Autodesk Fusion 360 part; units mm, degrees
(part 7 of 14)
  line L3871 (218.2079, 114.3) -> (223.7072, 123.825)
  line L3872 (237.4553, 144.4625) -> (226.4568, 144.4625)
  line L3873 (226.4568, 144.4625) -> (220.9575, 134.9375)
  line L3874 (220.9575, 134.9375) -> (226.4568, 125.4125)
  line L3875 (226.4568, 125.4125) -> (237.4553, 125.4125)
  line L3876 (242.9546, 134.9375) -> (237.4553, 144.4625)
  line L3877 (237.4553, 125.4125) -> (242.9546, 134.9375)
  line L3878 (256.7027, 155.575) -> (245.7042, 155.575)
  line L3879 (245.7042, 155.575) -> (240.2049, 146.05)
  line L3880 (240.2049, 146.05) -> (245.7042, 136.525)
  line L3881 (245.7042, 136.525) -> (256.7027, 136.525)
  line L3882 (262.202, 146.05) -> (256.7027, 155.575)
  line L3883 (256.7027, 136.525) -> (262.202, 146.05)
  line L3884 (275.9501, 166.6875) -> (264.9516, 166.6875)
  line L3885 (264.9516, 166.6875) -> (259.4524, 157.1625)
  line L3886 (259.4524, 157.1625) -> (264.9516, 147.6375)
  line L3887 (264.9516, 147.6375) -> (275.9501, 147.6375)
  line L3888 (281.4494, 157.1625) -> (275.9501, 166.6875)
  line L3889 (275.9501, 147.6375) -> (281.4494, 157.1625)
  line L3890 (295.1976, 177.8) -> (284.199, 177.8)
  line L3891 (284.199, 177.8) -> (278.6998, 168.275)
  line L3892 (278.6998, 168.275) -> (284.199, 158.75)
  line L3893 (284.199, 158.75) -> (295.1976, 158.75)
  line L3894 (300.6968, 168.275) -> (295.1976, 177.8)
  line L3895 (295.1976, 158.75) -> (300.6968, 168.275)
  line L3896 (314.445, 188.9125) -> (303.4464, 188.9125)
  line L3897 (303.4464, 188.9125) -> (297.9472, 179.3875)
  line L3898 (297.9472, 179.3875) -> (303.4464, 169.8625)
  line L3899 (303.4464, 169.8625) -> (314.445, 169.8625)
  line L3900 (319.9442, 179.3875) -> (314.445, 188.9125)
  line L3901 (314.445, 169.8625) -> (319.9442, 179.3875)
  line L3902 (333.6924, 200.025) -> (322.6939, 200.025)
  line L3903 (322.6939, 200.025) -> (317.1946, 190.5)
  line L3904 (317.1946, 190.5) -> (322.6939, 180.975)
  line L3905 (322.6939, 180.975) -> (333.6924, 180.975)
  line L3906 (339.1916, 190.5) -> (333.6924, 200.025)
  line L3907 (333.6924, 180.975) -> (339.1916, 190.5)
  line L3908 (352.9398, 211.1375) -> (341.9413, 211.1375)
  line L3909 (341.9413, 211.1375) -> (336.442, 201.6125)
  line L3910 (336.442, 201.6125) -> (341.9413, 192.0875)
  line L3911 (341.9413, 192.0875) -> (352.9398, 192.0875)
  line L3912 (358.4391, 201.6125) -> (352.9398, 211.1375)
  line L3913 (352.9398, 192.0875) -> (358.4391, 201.6125)
  line L3914 (372.1872, 222.25) -> (361.1887, 222.25)
  line L3915 (361.1887, 222.25) -> (355.6894, 212.725)
  line L3916 (355.6894, 212.725) -> (361.1887, 203.2)
  line L3917 (361.1887, 203.2) -> (372.1872, 203.2)
  line L3918 (377.6865, 212.725) -> (372.1872, 222.25)
  line L3919 (372.1872, 203.2) -> (377.6865, 212.725)
  line L3920 (391.4346, 233.3625) -> (380.4361, 233.3625)
  line L3921 (380.4361, 233.3625) -> (374.9368, 223.8375)
  line L3922 (374.9368, 223.8375) -> (380.4361, 214.3125)
  line L3923 (380.4361, 214.3125) -> (391.4346, 214.3125)
  line L3924 (396.9339, 223.8375) -> (391.4346, 233.3625)
  line L3925 (391.4346, 214.3125) -> (396.9339, 223.8375)
  line L3926 (410.682, 244.475) -> (399.6835, 244.475)
  line L3927 (399.6835, 244.475) -> (394.1843, 234.95)
  line L3928 (394.1843, 234.95) -> (399.6835, 225.425)
  line L3929 (399.6835, 225.425) -> (410.682, 225.425)
  line L3930 (416.1813, 234.95) -> (410.682, 244.475)
  line L3931 (410.682, 225.425) -> (416.1813, 234.95)
  line L3932 (429.9295, 255.5875) -> (418.9309, 255.5875)
  line L3933 (418.9309, 255.5875) -> (413.4317, 246.0625)
  line L3934 (413.4317, 246.0625) -> (418.9309, 236.5375)
  line L3935 (418.9309, 236.5375) -> (429.9295, 236.5375)
  line L3936 (435.4287, 246.0625) -> (429.9295, 255.5875)
  line L3937 (429.9295, 236.5375) -> (435.4287, 246.0625)
  line L3938 (449.1769, 266.7) -> (438.1783, 266.7)
  line L3939 (438.1783, 266.7) -> (432.6791, 257.175)
  line L3940 (432.6791, 257.175) -> (438.1783, 247.65)
  line L3941 (438.1783, 247.65) -> (449.1769, 247.65)
  line L3942 (454.6761, 257.175) -> (449.1769, 266.7)
  line L3943 (449.1769, 247.65) -> (454.6761, 257.175)
  line L3944 (468.4243, 277.8125) -> (457.4258, 277.8125)
  line L3945 (457.4258, 277.8125) -> (451.9265, 268.2875)
  line L3946 (451.9265, 268.2875) -> (457.4258, 258.7625)
  line L3947 (457.4258, 258.7625) -> (468.4243, 258.7625)
  line L3948 (473.9235, 268.2875) -> (468.4243, 277.8125)
  line L3949 (468.4243, 258.7625) -> (473.9235, 268.2875)
  line L3950 (487.6717, 288.925) -> (476.6732, 288.925)
  line L3951 (476.6732, 288.925) -> (471.1739, 279.4)
  line L3952 (471.1739, 279.4) -> (476.6732, 269.875)
  line L3953 (476.6732, 269.875) -> (487.6717, 269.875)
  line L3954 (493.171, 279.4) -> (487.6717, 288.925)
  line L3955 (487.6717, 269.875) -> (493.171, 279.4)
  line L3956 (506.9191, 300.0375) -> (495.9206, 300.0375)
  line L3957 (495.9206, 300.0375) -> (490.4213, 290.5125)
  line L3958 (490.4213, 290.5125) -> (495.9206, 280.9875)
  line L3959 (495.9206, 280.9875) -> (506.9191, 280.9875)
  line L3960 (512.4184, 290.5125) -> (506.9191, 300.0375)
  line L3961 (506.9191, 280.9875) -> (512.4184, 290.5125)
  line L3962 (526.1665, 311.15) -> (515.168, 311.15)
  line L3963 (515.168, 311.15) -> (509.6687, 301.625)
  line L3964 (509.6687, 301.625) -> (515.168, 292.1)
  line L3965 (515.168, 292.1) -> (526.1665, 292.1)
  line L3966 (531.6658, 301.625) -> (526.1665, 311.15)
  line L3967 (526.1665, 292.1) -> (531.6658, 301.625)
  line L3968 (545.4139, 322.2625) -> (534.4154, 322.2625)
  line L3969 (534.4154, 322.2625) -> (528.9162, 312.7375)
  line L3970 (528.9162, 312.7375) -> (534.4154, 303.2125)
  line L3971 (534.4154, 303.2125) -> (545.4139, 303.2125)
  line L3972 (550.9132, 312.7375) -> (545.4139, 322.2625)
  line L3973 (545.4139, 303.2125) -> (550.9132, 312.7375)
  line L3974 (564.6614, 333.375) -> (553.6628, 333.375)
  line L3975 (553.6628, 333.375) -> (548.1636, 323.85)
  line L3976 (548.1636, 323.85) -> (553.6628, 314.325)
  line L3977 (553.6628, 314.325) -> (564.6614, 314.325)
  line L3978 (570.1606, 323.85) -> (564.6614, 333.375)
  line L3979 (564.6614, 314.325) -> (570.1606, 323.85)
  line L3980 (-590.1835, -311.15) -> (-601.182, -311.15)
  line L3981 (-601.182, -311.15) -> (-606.6813, -320.675)
  line L3982 (-606.6813, -320.675) -> (-601.182, -330.2)
  line L3983 (-601.182, -330.2) -> (-590.1835, -330.2)
  line L3984 (-584.6843, -320.675) -> (-590.1835, -311.15)
  line L3985 (-590.1835, -330.2) -> (-584.6843, -320.675)
  line L3986 (-570.9361, -300.0375) -> (-581.9346, -300.0375)
  line L3987 (-581.9346, -300.0375) -> (-587.4339, -309.5625)
  line L3988 (-587.4339, -309.5625) -> (-581.9346, -319.0875)
  line L3989 (-581.9346, -319.0875) -> (-570.9361, -319.0875)
  line L3990 (-565.4368, -309.5625) -> (-570.9361, -300.0375)
  line L3991 (-570.9361, -319.0875) -> (-565.4368, -309.5625)
  line L3992 (-551.6887, -288.925) -> (-562.6872, -288.925)
  line L3993 (-562.6872, -288.925) -> (-568.1865, -298.45)
  line L3994 (-568.1865, -298.45) -> (-562.6872, -307.975)
  line L3995 (-562.6872, -307.975) -> (-551.6887, -307.975)
  line L3996 (-546.1894, -298.45) -> (-551.6887, -288.925)
  line L3997 (-551.6887, -307.975) -> (-546.1894, -298.45)
  line L3998 (-532.4413, -277.8125) -> (-543.4398, -277.8125)
  line L3999 (-543.4398, -277.8125) -> (-548.9391, -287.3375)
  line L4000 (-548.9391, -287.3375) -> (-543.4398, -296.8625)
  line L4001 (-543.4398, -296.8625) -> (-532.4413, -296.8625)
  line L4002 (-526.942, -287.3375) -> (-532.4413, -277.8125)
  line L4003 (-532.4413, -296.8625) -> (-526.942, -287.3375)
  line L4004 (-513.1939, -266.7) -> (-524.1924, -266.7)
  line L4005 (-524.1924, -266.7) -> (-529.6916, -276.225)
  line L4006 (-529.6916, -276.225) -> (-524.1924, -285.75)
  line L4007 (-524.1924, -285.75) -> (-513.1939, -285.75)
  line L4008 (-507.6946, -276.225) -> (-513.1939, -266.7)
  line L4009 (-513.1939, -285.75) -> (-507.6946, -276.225)
  line L4010 (-493.9464, -255.5875) -> (-504.945, -255.5875)
  line L4011 (-504.945, -255.5875) -> (-510.4442, -265.1125)
  line L4012 (-510.4442, -265.1125) -> (-504.945, -274.6375)
  line L4013 (-504.945, -274.6375) -> (-493.9464, -274.6375)
  line L4014 (-488.4472, -265.1125) -> (-493.9464, -255.5875)
  line L4015 (-493.9464, -274.6375) -> (-488.4472, -265.1125)
  line L4016 (-474.699, -244.475) -> (-485.6976, -244.475)
  line L4017 (-485.6976, -244.475) -> (-491.1968, -254)
  line L4018 (-491.1968, -254) -> (-485.6976, -263.525)
  line L4019 (-485.6976, -263.525) -> (-474.699, -263.525)
  line L4020 (-469.1998, -254) -> (-474.699, -244.475)
  line L4021 (-474.699, -263.525) -> (-469.1998, -254)
  line L4022 (-455.4516, -233.3625) -> (-466.4501, -233.3625)
  line L4023 (-466.4501, -233.3625) -> (-471.9494, -242.8875)
  line L4024 (-471.9494, -242.8875) -> (-466.4501, -252.4125)
  line L4025 (-466.4501, -252.4125) -> (-455.4516, -252.4125)
  line L4026 (-449.9524, -242.8875) -> (-455.4516, -233.3625)
  line L4027 (-455.4516, -252.4125) -> (-449.9524, -242.8875)
  line L4028 (-436.2042, -222.25) -> (-447.2027, -222.25)
  line L4029 (-447.2027, -222.25) -> (-452.702, -231.775)
  line L4030 (-452.702, -231.775) -> (-447.2027, -241.3)
  line L4031 (-447.2027, -241.3) -> (-436.2042, -241.3)
  line L4032 (-430.7049, -231.775) -> (-436.2042, -222.25)
  line L4033 (-436.2042, -241.3) -> (-430.7049, -231.775)
  line L4034 (-416.9568, -211.1375) -> (-427.9553, -211.1375)
  line L4035 (-427.9553, -211.1375) -> (-433.4546, -220.6625)
  line L4036 (-433.4546, -220.6625) -> (-427.9553, -230.1875)
  line L4037 (-427.9553, -230.1875) -> (-416.9568, -230.1875)
  line L4038 (-411.4575, -220.6625) -> (-416.9568, -211.1375)
  line L4039 (-416.9568, -230.1875) -> (-411.4575, -220.6625)
  line L4040 (-397.7094, -200.025) -> (-408.7079, -200.025)
  line L4041 (-408.7079, -200.025) -> (-414.2072, -209.55)
  line L4042 (-414.2072, -209.55) -> (-408.7079, -219.075)
  line L4043 (-408.7079, -219.075) -> (-397.7094, -219.075)
  line L4044 (-392.2101, -209.55) -> (-397.7094, -200.025)
  line L4045 (-397.7094, -219.075) -> (-392.2101, -209.55)
  line L4046 (-378.462, -188.9125) -> (-389.4605, -188.9125)
  line L4047 (-389.4605, -188.9125) -> (-394.9597, -198.4375)
  line L4048 (-394.9597, -198.4375) -> (-389.4605, -207.9625)
  line L4049 (-389.4605, -207.9625) -> (-378.462, -207.9625)
  line L4050 (-372.9627, -198.4375) -> (-378.462, -188.9125)
  line L4051 (-378.462, -207.9625) -> (-372.9627, -198.4375)
  line L4052 (-359.2145, -177.8) -> (-370.2131, -177.8)
  line L4053 (-370.2131, -177.8) -> (-375.7123, -187.325)
  line L4054 (-375.7123, -187.325) -> (-370.2131, -196.85)
  line L4055 (-370.2131, -196.85) -> (-359.2145, -196.85)
  line L4056 (-353.7153, -187.325) -> (-359.2145, -177.8)
  line L4057 (-359.2145, -196.85) -> (-353.7153, -187.325)
  line L4058 (-339.9671, -166.6875) -> (-350.9657, -166.6875)
  line L4059 (-350.9657, -166.6875) -> (-356.4649, -176.2125)
  line L4060 (-356.4649, -176.2125) -> (-350.9657, -185.7375)
  line L4061 (-350.9657, -185.7375) -> (-339.9671, -185.7375)
  line L4062 (-334.4679, -176.2125) -> (-339.9671, -166.6875)
  line L4063 (-339.9671, -185.7375) -> (-334.4679, -176.2125)
  line L4064 (-320.7197, -155.575) -> (-331.7182, -155.575)
  line L4065 (-331.7182, -155.575) -> (-337.2175, -165.1)
  line L4066 (-337.2175, -165.1) -> (-331.7182, -174.625)
  line L4067 (-331.7182, -174.625) -> (-320.7197, -174.625)
  line L4068 (-315.2205, -165.1) -> (-320.7197, -155.575)
  line L4069 (-320.7197, -174.625) -> (-315.2205, -165.1)
  line L4070 (-301.4723, -144.4625) -> (-312.4708, -144.4625)
  line L4071 (-312.4708, -144.4625) -> (-317.9701, -153.9875)
  line L4072 (-317.9701, -153.9875) -> (-312.4708, -163.5125)
  line L4073 (-312.4708, -163.5125) -> (-301.4723, -163.5125)
  line L4074 (-295.973, -153.9875) -> (-301.4723, -144.4625)
  line L4075 (-301.4723, -163.5125) -> (-295.973, -153.9875)
  line L4076 (-282.2249, -133.35) -> (-293.2234, -133.35)
  line L4077 (-293.2234, -133.35) -> (-298.7227, -142.875)
  line L4078 (-298.7227, -142.875) -> (-293.2234, -152.4)
  line L4079 (-293.2234, -152.4) -> (-282.2249, -152.4)
  line L4080 (-276.7256, -142.875) -> (-282.2249, -133.35)
  line L4081 (-282.2249, -152.4) -> (-276.7256, -142.875)
  line L4082 (-262.9775, -122.2375) -> (-273.976, -122.2375)
  line L4083 (-273.976, -122.2375) -> (-279.4753, -131.7625)
  line L4084 (-279.4753, -131.7625) -> (-273.976, -141.2875)
  line L4085 (-273.976, -141.2875) -> (-262.9775, -141.2875)
  line L4086 (-257.4782, -131.7625) -> (-262.9775, -122.2375)
  line L4087 (-262.9775, -141.2875) -> (-257.4782, -131.7625)
  line L4088 (-243.7301, -111.125) -> (-254.7286, -111.125)
  line L4089 (-254.7286, -111.125) -> (-260.2278, -120.65)
  line L4090 (-260.2278, -120.65) -> (-254.7286, -130.175)
  line L4091 (-254.7286, -130.175) -> (-243.7301, -130.175)
  line L4092 (-238.2308, -120.65) -> (-243.7301, -111.125)
  line L4093 (-243.7301, -130.175) -> (-238.2308, -120.65)
  line L4094 (-224.4826, -100.0125) -> (-235.4812, -100.0125)
  line L4095 (-235.4812, -100.0125) -> (-240.9804, -109.5375)
  line L4096 (-240.9804, -109.5375) -> (-235.4812, -119.0625)
  line L4097 (-235.4812, -119.0625) -> (-224.4826, -119.0625)
  line L4098 (-218.9834, -109.5375) -> (-224.4826, -100.0125)
  line L4099 (-224.4826, -119.0625) -> (-218.9834, -109.5375)
  line L4100 (-205.2352, -88.9) -> (-216.2337, -88.9)
  line L4101 (-216.2337, -88.9) -> (-221.733, -98.425)
  line L4102 (-221.733, -98.425) -> (-216.2337, -107.95)
  line L4103 (-216.2337, -107.95) -> (-205.2352, -107.95)
  line L4104 (-199.736, -98.425) -> (-205.2352, -88.9)
  line L4105 (-205.2352, -107.95) -> (-199.736, -98.425)
  line L4106 (-185.9878, -77.7875) -> (-196.9863, -77.7875)
  line L4107 (-196.9863, -77.7875) -> (-202.4856, -87.3125)
  line L4108 (-202.4856, -87.3125) -> (-196.9863, -96.8375)
  line L4109 (-196.9863, -96.8375) -> (-185.9878, -96.8375)
  line L4110 (-180.4886, -87.3125) -> (-185.9878, -77.7875)
  line L4111 (-185.9878, -96.8375) -> (-180.4886, -87.3125)
  line L4112 (-166.7404, -66.675) -> (-177.7389, -66.675)
  line L4113 (-177.7389, -66.675) -> (-183.2382, -76.2)
  line L4114 (-183.2382, -76.2) -> (-177.7389, -85.725)
  line L4115 (-177.7389, -85.725) -> (-166.7404, -85.725)
  line L4116 (-161.2411, -76.2) -> (-166.7404, -66.675)
  line L4117 (-166.7404, -85.725) -> (-161.2411, -76.2)
  line L4118 (-147.493, -55.5625) -> (-158.4915, -55.5625)
  line L4119 (-158.4915, -55.5625) -> (-163.9908, -65.0875)
  line L4120 (-163.9908, -65.0875) -> (-158.4915, -74.6125)
  line L4121 (-158.4915, -74.6125) -> (-147.493, -74.6125)
  line L4122 (-141.9937, -65.0875) -> (-147.493, -55.5625)
  line L4123 (-147.493, -74.6125) -> (-141.9937, -65.0875)
  line L4124 (-128.2456, -44.45) -> (-139.2441, -44.45)
  line L4125 (-139.2441, -44.45) -> (-144.7434, -53.975)
  line L4126 (-144.7434, -53.975) -> (-139.2441, -63.5)
  line L4127 (-139.2441, -63.5) -> (-128.2456, -63.5)
  line L4128 (-122.7463, -53.975) -> (-128.2456, -44.45)
  line L4129 (-128.2456, -63.5) -> (-122.7463, -53.975)
  line L4130 (-108.9982, -33.3375) -> (-119.9967, -33.3375)
  line L4131 (-119.9967, -33.3375) -> (-125.4959, -42.8625)
  line L4132 (-125.4959, -42.8625) -> (-119.9967, -52.3875)
  line L4133 (-119.9967, -52.3875) -> (-108.9982, -52.3875)
  line L4134 (-103.4989, -42.8625) -> (-108.9982, -33.3375)
  line L4135 (-108.9982, -52.3875) -> (-103.4989, -42.8625)
  line L4136 (-89.7507, -22.225) -> (-100.7493, -22.225)
  line L4137 (-100.7493, -22.225) -> (-106.2485, -31.75)
  line L4138 (-106.2485, -31.75) -> (-100.7493, -41.275)
  line L4139 (-100.7493, -41.275) -> (-89.7507, -41.275)
  line L4140 (-84.2515, -31.75) -> (-89.7507, -22.225)
  line L4141 (-89.7507, -41.275) -> (-84.2515, -31.75)
  line L4142 (-70.5033, -11.1125) -> (-81.5018, -11.1125)
  line L4143 (-81.5018, -11.1125) -> (-87.0011, -20.6375)
  line L4144 (-87.0011, -20.6375) -> (-81.5018, -30.1625)
  line L4145 (-81.5018, -30.1625) -> (-70.5033, -30.1625)
  line L4146 (-65.0041, -20.6375) -> (-70.5033, -11.1125)
  line L4147 (-70.5033, -30.1625) -> (-65.0041, -20.6375)
  line L4148 (-51.2559, 0) -> (-62.2544, 0)
  line L4149 (-62.2544, 0) -> (-67.7537, -9.525)
  line L4150 (-67.7537, -9.525) -> (-62.2544, -19.05)
  line L4151 (-62.2544, -19.05) -> (-51.2559, -19.05)
  line L4152 (-45.7566, -9.525) -> (-51.2559, 0)
  line L4153 (-51.2559, -19.05) -> (-45.7566, -9.525)
  line L4154 (-32.0085, 11.1125) -> (-43.007, 11.1125)
  line L4155 (-43.007, 11.1125) -> (-48.5063, 1.5875)
  line L4156 (-48.5063, 1.5875) -> (-43.007, -7.9375)
  line L4157 (-43.007, -7.9375) -> (-32.0085, -7.9375)
  line L4158 (-26.5092, 1.5875) -> (-32.0085, 11.1125)
  line L4159 (-32.0085, -7.9375) -> (-26.5092, 1.5875)
  line L4160 (-12.7611, 22.225) -> (-23.7596, 22.225)
  line L4161 (-23.7596, 22.225) -> (-29.2589, 12.7)
  line L4162 (-29.2589, 12.7) -> (-23.7596, 3.175)
  line L4163 (-23.7596, 3.175) -> (-12.7611, 3.175)
  line L4164 (-7.2618, 12.7) -> (-12.7611, 22.225)
  line L4165 (-12.7611, 3.175) -> (-7.2618, 12.7)
  line L4166 (6.4863, 33.3375) -> (-4.5122, 33.3375)
  line L4167 (-4.5122, 33.3375) -> (-10.0114, 23.8125)
  line L4168 (-10.0114, 23.8125) -> (-4.5122, 14.2875)
  line L4169 (-4.5122, 14.2875) -> (6.4863, 14.2875)
  line L4170 (11.9856, 23.8125) -> (6.4863, 33.3375)
  line L4171 (6.4863, 14.2875) -> (11.9856, 23.8125)
  line L4172 (25.7337, 44.45) -> (14.7352, 44.45)
  line L4173 (14.7352, 44.45) -> (9.236, 34.925)
  line L4174 (9.236, 34.925) -> (14.7352, 25.4)
  line L4175 (14.7352, 25.4) -> (25.7337, 25.4)
  line L4176 (31.233, 34.925) -> (25.7337, 44.45)
  line L4177 (25.7337, 25.4) -> (31.233, 34.925)
  line L4178 (44.9812, 55.5625) -> (33.9826, 55.5625)
  line L4179 (33.9826, 55.5625) -> (28.4834, 46.0375)
  line L4180 (28.4834, 46.0375) -> (33.9826, 36.5125)
  line L4181 (33.9826, 36.5125) -> (44.9812, 36.5125)
  line L4182 (50.4804, 46.0375) -> (44.9812, 55.5625)
  line L4183 (44.9812, 36.5125) -> (50.4804, 46.0375)
  line L4184 (64.2286, 66.675) -> (53.2301, 66.675)
  line L4185 (53.2301, 66.675) -> (47.7308, 57.15)
  line L4186 (47.7308, 57.15) -> (53.2301, 47.625)
  line L4187 (53.2301, 47.625) -> (64.2286, 47.625)
  line L4188 (69.7278, 57.15) -> (64.2286, 66.675)
  line L4189 (64.2286, 47.625) -> (69.7278, 57.15)
  line L4190 (83.476, 77.7875) -> (72.4775, 77.7875)
  line L4191 (72.4775, 77.7875) -> (66.9782, 68.2625)
  line L4192 (66.9782, 68.2625) -> (72.4775, 58.7375)
  line L4193 (72.4775, 58.7375) -> (83.476, 58.7375)
  line L4194 (88.9753, 68.2625) -> (83.476, 77.7875)
  line L4195 (83.476, 58.7375) -> (88.9753, 68.2625)
  line L4196 (102.7234, 88.9) -> (91.7249, 88.9)
  line L4197 (91.7249, 88.9) -> (86.2256, 79.375)
  line L4198 (86.2256, 79.375) -> (91.7249, 69.85)
  line L4199 (91.7249, 69.85) -> (102.7234, 69.85)
  line L4200 (108.2227, 79.375) -> (102.7234, 88.9)
  line L4201 (102.7234, 69.85) -> (108.2227, 79.375)
  line L4202 (121.9708, 100.0125) -> (110.9723, 100.0125)
  line L4203 (110.9723, 100.0125) -> (105.473, 90.4875)
  line L4204 (105.473, 90.4875) -> (110.9723, 80.9625)
  line L4205 (110.9723, 80.9625) -> (121.9708, 80.9625)
  line L4206 (127.4701, 90.4875) -> (121.9708, 100.0125)
  line L4207 (121.9708, 80.9625) -> (127.4701, 90.4875)
  line L4208 (141.2182, 111.125) -> (130.2197, 111.125)
  line L4209 (130.2197, 111.125) -> (124.7205, 101.6)
  line L4210 (124.7205, 101.6) -> (130.2197, 92.075)
  line L4211 (130.2197, 92.075) -> (141.2182, 92.075)
  line L4212 (146.7175, 101.6) -> (141.2182, 111.125)
  line L4213 (141.2182, 92.075) -> (146.7175, 101.6)
  line L4214 (160.4657, 122.2375) -> (149.4671, 122.2375)
  line L4215 (149.4671, 122.2375) -> (143.9679, 112.7125)
  line L4216 (143.9679, 112.7125) -> (149.4671, 103.1875)
  line L4217 (149.4671, 103.1875) -> (160.4657, 103.1875)
  line L4218 (165.9649, 112.7125) -> (160.4657, 122.2375)
  line L4219 (160.4657, 103.1875) -> (165.9649, 112.7125)
  line L4220 (179.7131, 133.35) -> (168.7145, 133.35)
  line L4221 (168.7145, 133.35) -> (163.2153, 123.825)
  line L4222 (163.2153, 123.825) -> (168.7145, 114.3)
  line L4223 (168.7145, 114.3) -> (179.7131, 114.3)
  line L4224 (185.2123, 123.825) -> (179.7131, 133.35)
  line L4225 (179.7131, 114.3) -> (185.2123, 123.825)
  line L4226 (198.9605, 144.4625) -> (187.962, 144.4625)
  line L4227 (187.962, 144.4625) -> (182.4627, 134.9375)
  line L4228 (182.4627, 134.9375) -> (187.962, 125.4125)
  line L4229 (187.962, 125.4125) -> (198.9605, 125.4125)
  line L4230 (204.4597, 134.9375) -> (198.9605, 144.4625)
  line L4231 (198.9605, 125.4125) -> (204.4597, 134.9375)
  line L4232 (218.2079, 155.575) -> (207.2094, 155.575)
  line L4233 (207.2094, 155.575) -> (201.7101, 146.05)
  line L4234 (201.7101, 146.05) -> (207.2094, 136.525)
  line L4235 (207.2094, 136.525) -> (218.2079, 136.525)
  line L4236 (223.7072, 146.05) -> (218.2079, 155.575)
  line L4237 (218.2079, 136.525) -> (223.7072, 146.05)
  line L4238 (237.4553, 166.6875) -> (226.4568, 166.6875)
  line L4239 (226.4568, 166.6875) -> (220.9575, 157.1625)
  line L4240 (220.9575, 157.1625) -> (226.4568, 147.6375)
  line L4241 (226.4568, 147.6375) -> (237.4553, 147.6375)
  line L4242 (242.9546, 157.1625) -> (237.4553, 166.6875)
  line L4243 (237.4553, 147.6375) -> (242.9546, 157.1625)
  line L4244 (256.7027, 177.8) -> (245.7042, 177.8)
  line L4245 (245.7042, 177.8) -> (240.2049, 168.275)
  line L4246 (240.2049, 168.275) -> (245.7042, 158.75)
  line L4247 (245.7042, 158.75) -> (256.7027, 158.75)
  line L4248 (262.202, 168.275) -> (256.7027, 177.8)
  line L4249 (256.7027, 158.75) -> (262.202, 168.275)
  line L4250 (275.9501, 188.9125) -> (264.9516, 188.9125)
  line L4251 (264.9516, 188.9125) -> (259.4524, 179.3875)
  line L4252 (259.4524, 179.3875) -> (264.9516, 169.8625)
  line L4253 (264.9516, 169.8625) -> (275.9501, 169.8625)
  line L4254 (281.4494, 179.3875) -> (275.9501, 188.9125)
  line L4255 (275.9501, 169.8625) -> (281.4494, 179.3875)
  line L4256 (295.1976, 200.025) -> (284.199, 200.025)
  line L4257 (284.199, 200.025) -> (278.6998, 190.5)
  line L4258 (278.6998, 190.5) -> (284.199, 180.975)
  line L4259 (284.199, 180.975) -> (295.1976, 180.975)
  line L4260 (300.6968, 190.5) -> (295.1976, 200.025)
  line L4261 (295.1976, 180.975) -> (300.6968, 190.5)
  line L4262 (314.445, 211.1375) -> (303.4464, 211.1375)
  line L4263 (303.4464, 211.1375) -> (297.9472, 201.6125)
  line L4264 (297.9472, 201.6125) -> (303.4464, 192.0875)
  line L4265 (303.4464, 192.0875) -> (314.445, 192.0875)
  line L4266 (319.9442, 201.6125) -> (314.445, 211.1375)
  line L4267 (314.445, 192.0875) -> (319.9442, 201.6125)
  line L4268 (333.6924, 222.25) -> (322.6939, 222.25)
  line L4269 (322.6939, 222.25) -> (317.1946, 212.725)
  line L4270 (317.1946, 212.725) -> (322.6939, 203.2)
  line L4271 (322.6939, 203.2) -> (333.6924, 203.2)
  line L4272 (339.1916, 212.725) -> (333.6924, 222.25)
  line L4273 (333.6924, 203.2) -> (339.1916, 212.725)
  line L4274 (352.9398, 233.3625) -> (341.9413, 233.3625)
  line L4275 (341.9413, 233.3625) -> (336.442, 223.8375)
  line L4276 (336.442, 223.8375) -> (341.9413, 214.3125)
  line L4277 (341.9413, 214.3125) -> (352.9398, 214.3125)
  line L4278 (358.4391, 223.8375) -> (352.9398, 233.3625)
  line L4279 (352.9398, 214.3125) -> (358.4391, 223.8375)
  line L4280 (372.1872, 244.475) -> (361.1887, 244.475)
  line L4281 (361.1887, 244.475) -> (355.6894, 234.95)
  line L4282 (355.6894, 234.95) -> (361.1887, 225.425)
  line L4283 (361.1887, 225.425) -> (372.1872, 225.425)
  line L4284 (377.6865, 234.95) -> (372.1872, 244.475)
  line L4285 (372.1872, 225.425) -> (377.6865, 234.95)
  line L4286 (391.4346, 255.5875) -> (380.4361, 255.5875)
  line L4287 (380.4361, 255.5875) -> (374.9368, 246.0625)
  line L4288 (374.9368, 246.0625) -> (380.4361, 236.5375)
  line L4289 (380.4361, 236.5375) -> (391.4346, 236.5375)
  line L4290 (396.9339, 246.0625) -> (391.4346, 255.5875)
  line L4291 (391.4346, 236.5375) -> (396.9339, 246.0625)
  line L4292 (410.682, 266.7) -> (399.6835, 266.7)
  line L4293 (399.6835, 266.7) -> (394.1843, 257.175)
  line L4294 (394.1843, 257.175) -> (399.6835, 247.65)
  line L4295 (399.6835, 247.65) -> (410.682, 247.65)
  line L4296 (416.1813, 257.175) -> (410.682, 266.7)
  line L4297 (410.682, 247.65) -> (416.1813, 257.175)
  line L4298 (429.9295, 277.8125) -> (418.9309, 277.8125)
  line L4299 (418.9309, 277.8125) -> (413.4317, 268.2875)
  line L4300 (413.4317, 268.2875) -> (418.9309, 258.7625)
  line L4301 (418.9309, 258.7625) -> (429.9295, 258.7625)
  line L4302 (435.4287, 268.2875) -> (429.9295, 277.8125)
  line L4303 (429.9295, 258.7625) -> (435.4287, 268.2875)
  line L4304 (449.1769, 288.925) -> (438.1783, 288.925)
  line L4305 (438.1783, 288.925) -> (432.6791, 279.4)
  line L4306 (432.6791, 279.4) -> (438.1783, 269.875)
  line L4307 (438.1783, 269.875) -> (449.1769, 269.875)
  line L4308 (454.6761, 279.4) -> (449.1769, 288.925)
  line L4309 (449.1769, 269.875) -> (454.6761, 279.4)
  line L4310 (468.4243, 300.0375) -> (457.4258, 300.0375)
  line L4311 (457.4258, 300.0375) -> (451.9265, 290.5125)
  line L4312 (451.9265, 290.5125) -> (457.4258, 280.9875)
  line L4313 (457.4258, 280.9875) -> (468.4243, 280.9875)
  line L4314 (473.9235, 290.5125) -> (468.4243, 300.0375)
  line L4315 (468.4243, 280.9875) -> (473.9235, 290.5125)
  line L4316 (487.6717, 311.15) -> (476.6732, 311.15)
  line L4317 (476.6732, 311.15) -> (471.1739, 301.625)
  line L4318 (471.1739, 301.625) -> (476.6732, 292.1)
  line L4319 (476.6732, 292.1) -> (487.6717, 292.1)
  line L4320 (493.171, 301.625) -> (487.6717, 311.15)
  line L4321 (487.6717, 292.1) -> (493.171, 301.625)
  line L4322 (506.9191, 322.2625) -> (495.9206, 322.2625)
  line L4323 (495.9206, 322.2625) -> (490.4213, 312.7375)
  line L4324 (490.4213, 312.7375) -> (495.9206, 303.2125)
  line L4325 (495.9206, 303.2125) -> (506.9191, 303.2125)
  line L4326 (512.4184, 312.7375) -> (506.9191, 322.2625)
  line L4327 (506.9191, 303.2125) -> (512.4184, 312.7375)
  line L4328 (526.1665, 333.375) -> (515.168, 333.375)
  line L4329 (515.168, 333.375) -> (509.6687, 323.85)
  line L4330 (509.6687, 323.85) -> (515.168, 314.325)
  line L4331 (515.168, 314.325) -> (526.1665, 314.325)
  line L4332 (531.6658, 323.85) -> (526.1665, 333.375)
  line L4333 (526.1665, 314.325) -> (531.6658, 323.85)
  line L4334 (545.4139, 344.4875) -> (534.4154, 344.4875)
  line L4335 (534.4154, 344.4875) -> (528.9162, 334.9625)
  line L4336 (528.9162, 334.9625) -> (534.4154, 325.4375)
  line L4337 (534.4154, 325.4375) -> (545.4139, 325.4375)
  line L4338 (550.9132, 334.9625) -> (545.4139, 344.4875)
  line L4339 (545.4139, 325.4375) -> (550.9132, 334.9625)
  line L4340 (-609.4309, -300.0375) -> (-620.4295, -300.0375)
  line L4341 (-620.4295, -300.0375) -> (-625.9287, -309.5625)
  line L4342 (-625.9287, -309.5625) -> (-620.4295, -319.0875)
  line L4343 (-620.4295, -319.0875) -> (-609.4309, -319.0875)
  line L4344 (-603.9317, -309.5625) -> (-609.4309, -300.0375)
  line L4345 (-609.4309, -319.0875) -> (-603.9317, -309.5625)
  line L4346 (-590.1835, -288.925) -> (-601.182, -288.925)
  line L4347 (-601.182, -288.925) -> (-606.6813, -298.45)
  line L4348 (-606.6813, -298.45) -> (-601.182, -307.975)
  line L4349 (-601.182, -307.975) -> (-590.1835, -307.975)
  line L4350 (-584.6843, -298.45) -> (-590.1835, -288.925)
  line L4351 (-590.1835, -307.975) -> (-584.6843, -298.45)
  line L4352 (-570.9361, -277.8125) -> (-581.9346, -277.8125)
  line L4353 (-581.9346, -277.8125) -> (-587.4339, -287.3375)
  line L4354 (-587.4339, -287.3375) -> (-581.9346, -296.8625)
  line L4355 (-581.9346, -296.8625) -> (-570.9361, -296.8625)
  line L4356 (-565.4368, -287.3375) -> (-570.9361, -277.8125)
  line L4357 (-570.9361, -296.8625) -> (-565.4368, -287.3375)
  line L4358 (-551.6887, -266.7) -> (-562.6872, -266.7)
  line L4359 (-562.6872, -266.7) -> (-568.1865, -276.225)
  line L4360 (-568.1865, -276.225) -> (-562.6872, -285.75)
  line L4361 (-562.6872, -285.75) -> (-551.6887, -285.75)
  line L4362 (-546.1894, -276.225) -> (-551.6887, -266.7)
  line L4363 (-551.6887, -285.75) -> (-546.1894, -276.225)
  line L4364 (-532.4413, -255.5875) -> (-543.4398, -255.5875)
  line L4365 (-543.4398, -255.5875) -> (-548.9391, -265.1125)
  line L4366 (-548.9391, -265.1125) -> (-543.4398, -274.6375)
  line L4367 (-543.4398, -274.6375) -> (-532.4413, -274.6375)
  line L4368 (-526.942, -265.1125) -> (-532.4413, -255.5875)
  line L4369 (-532.4413, -274.6375) -> (-526.942, -265.1125)
  line L4370 (-513.1939, -244.475) -> (-524.1924, -244.475)
  line L4371 (-524.1924, -244.475) -> (-529.6916, -254)
  line L4372 (-529.6916, -254) -> (-524.1924, -263.525)
  line L4373 (-524.1924, -263.525) -> (-513.1939, -263.525)
  line L4374 (-507.6946, -254) -> (-513.1939, -244.475)
  line L4375 (-513.1939, -263.525) -> (-507.6946, -254)
  line L4376 (-493.9464, -233.3625) -> (-504.945, -233.3625)
  line L4377 (-504.945, -233.3625) -> (-510.4442, -242.8875)
  line L4378 (-510.4442, -242.8875) -> (-504.945, -252.4125)
  line L4379 (-504.945, -252.4125) -> (-493.9464, -252.4125)
  line L4380 (-488.4472, -242.8875) -> (-493.9464, -233.3625)
  line L4381 (-493.9464, -252.4125) -> (-488.4472, -242.8875)
  line L4382 (-474.699, -222.25) -> (-485.6976, -222.25)
  line L4383 (-485.6976, -222.25) -> (-491.1968, -231.775)
  line L4384 (-491.1968, -231.775) -> (-485.6976, -241.3)
  line L4385 (-485.6976, -241.3) -> (-474.699, -241.3)
  line L4386 (-469.1998, -231.775) -> (-474.699, -222.25)
  line L4387 (-474.699, -241.3) -> (-469.1998, -231.775)
  line L4388 (-455.4516, -211.1375) -> (-466.4501, -211.1375)
  line L4389 (-466.4501, -211.1375) -> (-471.9494, -220.6625)
  line L4390 (-471.9494, -220.6625) -> (-466.4501, -230.1875)
  line L4391 (-466.4501, -230.1875) -> (-455.4516, -230.1875)
  line L4392 (-449.9524, -220.6625) -> (-455.4516, -211.1375)
  line L4393 (-455.4516, -230.1875) -> (-449.9524, -220.6625)
  line L4394 (-436.2042, -200.025) -> (-447.2027, -200.025)
  line L4395 (-447.2027, -200.025) -> (-452.702, -209.55)
  line L4396 (-452.702, -209.55) -> (-447.2027, -219.075)
  line L4397 (-447.2027, -219.075) -> (-436.2042, -219.075)
  line L4398 (-430.7049, -209.55) -> (-436.2042, -200.025)
  line L4399 (-436.2042, -219.075) -> (-430.7049, -209.55)
  line L4400 (-416.9568, -188.9125) -> (-427.9553, -188.9125)
  line L4401 (-427.9553, -188.9125) -> (-433.4546, -198.4375)
  line L4402 (-433.4546, -198.4375) -> (-427.9553, -207.9625)
  line L4403 (-427.9553, -207.9625) -> (-416.9568, -207.9625)
  line L4404 (-411.4575, -198.4375) -> (-416.9568, -188.9125)
  line L4405 (-416.9568, -207.9625) -> (-411.4575, -198.4375)
  line L4406 (-397.7094, -177.8) -> (-408.7079, -177.8)
  line L4407 (-408.7079, -177.8) -> (-414.2072, -187.325)
  line L4408 (-414.2072, -187.325) -> (-408.7079, -196.85)
  line L4409 (-408.7079, -196.85) -> (-397.7094, -196.85)
  line L4410 (-392.2101, -187.325) -> (-397.7094, -177.8)
  line L4411 (-397.7094, -196.85) -> (-392.2101, -187.325)
  line L4412 (-378.462, -166.6875) -> (-389.4605, -166.6875)
  line L4413 (-389.4605, -166.6875) -> (-394.9597, -176.2125)
  line L4414 (-394.9597, -176.2125) -> (-389.4605, -185.7375)
  line L4415 (-389.4605, -185.7375) -> (-378.462, -185.7375)
  line L4416 (-372.9627, -176.2125) -> (-378.462, -166.6875)
  line L4417 (-378.462, -185.7375) -> (-372.9627, -176.2125)
  line L4418 (-359.2145, -155.575) -> (-370.2131, -155.575)
  line L4419 (-370.2131, -155.575) -> (-375.7123, -165.1)
  line L4420 (-375.7123, -165.1) -> (-370.2131, -174.625)
  line L4421 (-370.2131, -174.625) -> (-359.2145, -174.625)
  line L4422 (-353.7153, -165.1) -> (-359.2145, -155.575)
  line L4423 (-359.2145, -174.625) -> (-353.7153, -165.1)
  line L4424 (-339.9671, -144.4625) -> (-350.9657, -144.4625)
  line L4425 (-350.9657, -144.4625) -> (-356.4649, -153.9875)
  line L4426 (-356.4649, -153.9875) -> (-350.9657, -163.5125)
  line L4427 (-350.9657, -163.5125) -> (-339.9671, -163.5125)
  line L4428 (-334.4679, -153.9875) -> (-339.9671, -144.4625)
  line L4429 (-339.9671, -163.5125) -> (-334.4679, -153.9875)
  line L4430 (-320.7197, -133.35) -> (-331.7182, -133.35)
  line L4431 (-331.7182, -133.35) -> (-337.2175, -142.875)
  line L4432 (-337.2175, -142.875) -> (-331.7182, -152.4)
  line L4433 (-331.7182, -152.4) -> (-320.7197, -152.4)
  line L4434 (-315.2205, -142.875) -> (-320.7197, -133.35)
  line L4435 (-320.7197, -152.4) -> (-315.2205, -142.875)
  line L4436 (-301.4723, -122.2375) -> (-312.4708, -122.2375)
  line L4437 (-312.4708, -122.2375) -> (-317.9701, -131.7625)
  line L4438 (-317.9701, -131.7625) -> (-312.4708, -141.2875)
  line L4439 (-312.4708, -141.2875) -> (-301.4723, -141.2875)
  line L4440 (-295.973, -131.7625) -> (-301.4723, -122.2375)
  line L4441 (-301.4723, -141.2875) -> (-295.973, -131.7625)
  line L4442 (-282.2249, -111.125) -> (-293.2234, -111.125)
  line L4443 (-293.2234, -111.125) -> (-298.7227, -120.65)
  line L4444 (-298.7227, -120.65) -> (-293.2234, -130.175)
  line L4445 (-293.2234, -130.175) -> (-282.2249, -130.175)
  line L4446 (-276.7256, -120.65) -> (-282.2249, -111.125)
  line L4447 (-282.2249, -130.175) -> (-276.7256, -120.65)
  line L4448 (-262.9775, -100.0125) -> (-273.976, -100.0125)
  line L4449 (-273.976, -100.0125) -> (-279.4753, -109.5375)
  line L4450 (-279.4753, -109.5375) -> (-273.976, -119.0625)
  line L4451 (-273.976, -119.0625) -> (-262.9775, -119.0625)
  line L4452 (-257.4782, -109.5375) -> (-262.9775, -100.0125)
  line L4453 (-262.9775, -119.0625) -> (-257.4782, -109.5375)
  line L4454 (-243.7301, -88.9) -> (-254.7286, -88.9)
  line L4455 (-254.7286, -88.9) -> (-260.2278, -98.425)
  line L4456 (-260.2278, -98.425) -> (-254.7286, -107.95)
  line L4457 (-254.7286, -107.95) -> (-243.7301, -107.95)
  line L4458 (-238.2308, -98.425) -> (-243.7301, -88.9)
  line L4459 (-243.7301, -107.95) -> (-238.2308, -98.425)
  line L4460 (-224.4826, -77.7875) -> (-235.4812, -77.7875)
  line L4461 (-235.4812, -77.7875) -> (-240.9804, -87.3125)
  line L4462 (-240.9804, -87.3125) -> (-235.4812, -96.8375)
  line L4463 (-235.4812, -96.8375) -> (-224.4826, -96.8375)
  line L4464 (-218.9834, -87.3125) -> (-224.4826, -77.7875)
  line L4465 (-224.4826, -96.8375) -> (-218.9834, -87.3125)
  line L4466 (-205.2352, -66.675) -> (-216.2337, -66.675)
  line L4467 (-216.2337, -66.675) -> (-221.733, -76.2)
  line L4468 (-221.733, -76.2) -> (-216.2337, -85.725)
  line L4469 (-216.2337, -85.725) -> (-205.2352, -85.725)
  line L4470 (-199.736, -76.2) -> (-205.2352, -66.675)
  line L4471 (-205.2352, -85.725) -> (-199.736, -76.2)
  line L4472 (-185.9878, -55.5625) -> (-196.9863, -55.5625)
  line L4473 (-196.9863, -55.5625) -> (-202.4856, -65.0875)
  line L4474 (-202.4856, -65.0875) -> (-196.9863, -74.6125)
  line L4475 (-196.9863, -74.6125) -> (-185.9878, -74.6125)
  line L4476 (-180.4886, -65.0875) -> (-185.9878, -55.5625)
  line L4477 (-185.9878, -74.6125) -> (-180.4886, -65.0875)
  line L4478 (-166.7404, -44.45) -> (-177.7389, -44.45)
  line L4479 (-177.7389, -44.45) -> (-183.2382, -53.975)
  line L4480 (-183.2382, -53.975) -> (-177.7389, -63.5)
  line L4481 (-177.7389, -63.5) -> (-166.7404, -63.5)
  line L4482 (-161.2411, -53.975) -> (-166.7404, -44.45)
  line L4483 (-166.7404, -63.5) -> (-161.2411, -53.975)
  line L4484 (-147.493, -33.3375) -> (-158.4915, -33.3375)
  line L4485 (-158.4915, -33.3375) -> (-163.9908, -42.8625)
  line L4486 (-163.9908, -42.8625) -> (-158.4915, -52.3875)
  line L4487 (-158.4915, -52.3875) -> (-147.493, -52.3875)
  line L4488 (-141.9937, -42.8625) -> (-147.493, -33.3375)
  line L4489 (-147.493, -52.3875) -> (-141.9937, -42.8625)
  line L4490 (-128.2456, -22.225) -> (-139.2441, -22.225)
  line L4491 (-139.2441, -22.225) -> (-144.7434, -31.75)
  line L4492 (-144.7434, -31.75) -> (-139.2441, -41.275)
  line L4493 (-139.2441, -41.275) -> (-128.2456, -41.275)
  line L4494 (-122.7463, -31.75) -> (-128.2456, -22.225)
  line L4495 (-128.2456, -41.275) -> (-122.7463, -31.75)
  line L4496 (-108.9982, -11.1125) -> (-119.9967, -11.1125)
  line L4497 (-119.9967, -11.1125) -> (-125.4959, -20.6375)
  line L4498 (-125.4959, -20.6375) -> (-119.9967, -30.1625)
  line L4499 (-119.9967, -30.1625) -> (-108.9982, -30.1625)
  line L4500 (-103.4989, -20.6375) -> (-108.9982, -11.1125)
  line L4501 (-108.9982, -30.1625) -> (-103.4989, -20.6375)
  line L4502 (-89.7507, 0) -> (-100.7493, 0)
  line L4503 (-100.7493, 0) -> (-106.2485, -9.525)
  line L4504 (-106.2485, -9.525) -> (-100.7493, -19.05)
  line L4505 (-100.7493, -19.05) -> (-89.7507, -19.05)
  line L4506 (-84.2515, -9.525) -> (-89.7507, 0)
  line L4507 (-89.7507, -19.05) -> (-84.2515, -9.525)
  line L4508 (-70.5033, 11.1125) -> (-81.5018, 11.1125)
  line L4509 (-81.5018, 11.1125) -> (-87.0011, 1.5875)
  line L4510 (-87.0011, 1.5875) -> (-81.5018, -7.9375)
  line L4511 (-81.5018, -7.9375) -> (-70.5033, -7.9375)
  line L4512 (-65.0041, 1.5875) -> (-70.5033, 11.1125)
  line L4513 (-70.5033, -7.9375) -> (-65.0041, 1.5875)
  line L4514 (-51.2559, 22.225) -> (-62.2544, 22.225)
  line L4515 (-62.2544, 22.225) -> (-67.7537, 12.7)
  line L4516 (-67.7537, 12.7) -> (-62.2544, 3.175)
  line L4517 (-62.2544, 3.175) -> (-51.2559, 3.175)
  line L4518 (-45.7566, 12.7) -> (-51.2559, 22.225)
  line L4519 (-51.2559, 3.175) -> (-45.7566, 12.7)
  line L4520 (-32.0085, 33.3375) -> (-43.007, 33.3375)
  line L4521 (-43.007, 33.3375) -> (-48.5063, 23.8125)
  line L4522 (-48.5063, 23.8125) -> (-43.007, 14.2875)
  line L4523 (-43.007, 14.2875) -> (-32.0085, 14.2875)
  line L4524 (-26.5092, 23.8125) -> (-32.0085, 33.3375)
  line L4525 (-32.0085, 14.2875) -> (-26.5092, 23.8125)
  line L4526 (-12.7611, 44.45) -> (-23.7596, 44.45)
  line L4527 (-23.7596, 44.45) -> (-29.2589, 34.925)
  line L4528 (-29.2589, 34.925) -> (-23.7596, 25.4)
  line L4529 (-23.7596, 25.4) -> (-12.7611, 25.4)
  line L4530 (-7.2618, 34.925) -> (-12.7611, 44.45)
  line L4531 (-12.7611, 25.4) -> (-7.2618, 34.925)
  line L4532 (6.4863, 55.5625) -> (-4.5122, 55.5625)
  line L4533 (-4.5122, 55.5625) -> (-10.0114, 46.0375)
  line L4534 (-10.0114, 46.0375) -> (-4.5122, 36.5125)
  line L4535 (-4.5122, 36.5125) -> (6.4863, 36.5125)
  line L4536 (11.9856, 46.0375) -> (6.4863, 55.5625)
  line L4537 (6.4863, 36.5125) -> (11.9856, 46.0375)
  line L4538 (25.7337, 66.675) -> (14.7352, 66.675)
  line L4539 (14.7352, 66.675) -> (9.236, 57.15)
  line L4540 (9.236, 57.15) -> (14.7352, 47.625)
  line L4541 (14.7352, 47.625) -> (25.7337, 47.625)
  line L4542 (31.233, 57.15) -> (25.7337, 66.675)
  line L4543 (25.7337, 47.625) -> (31.233, 57.15)
  line L4544 (44.9812, 77.7875) -> (33.9826, 77.7875)
  line L4545 (33.9826, 77.7875) -> (28.4834, 68.2625)
  line L4546 (28.4834, 68.2625) -> (33.9826, 58.7375)
  line L4547 (33.9826, 58.7375) -> (44.9812, 58.7375)
  line L4548 (50.4804, 68.2625) -> (44.9812, 77.7875)
  line L4549 (44.9812, 58.7375) -> (50.4804, 68.2625)
  line L4550 (64.2286, 88.9) -> (53.2301, 88.9)
  line L4551 (53.2301, 88.9) -> (47.7308, 79.375)
  line L4552 (47.7308, 79.375) -> (53.2301, 69.85)
  line L4553 (53.2301, 69.85) -> (64.2286, 69.85)
  line L4554 (69.7278, 79.375) -> (64.2286, 88.9)
  line L4555 (64.2286, 69.85) -> (69.7278, 79.375)
  line L4556 (83.476, 100.0125) -> (72.4775, 100.0125)
  line L4557 (72.4775, 100.0125) -> (66.9782, 90.4875)
  line L4558 (66.9782, 90.4875) -> (72.4775, 80.9625)
  line L4559 (72.4775, 80.9625) -> (83.476, 80.9625)
  line L4560 (88.9753, 90.4875) -> (83.476, 100.0125)
  line L4561 (83.476, 80.9625) -> (88.9753, 90.4875)
  line L4562 (102.7234, 111.125) -> (91.7249, 111.125)
  line L4563 (91.7249, 111.125) -> (86.2256, 101.6)
  line L4564 (86.2256, 101.6) -> (91.7249, 92.075)
  line L4565 (91.7249, 92.075) -> (102.7234, 92.075)
  line L4566 (108.2227, 101.6) -> (102.7234, 111.125)
  line L4567 (102.7234, 92.075) -> (108.2227, 101.6)
  line L4568 (121.9708, 122.2375) -> (110.9723, 122.2375)
  line L4569 (110.9723, 122.2375) -> (105.473, 112.7125)
  line L4570 (105.473, 112.7125) -> (110.9723, 103.1875)
  line L4571 (110.9723, 103.1875) -> (121.9708, 103.1875)
  line L4572 (127.4701, 112.7125) -> (121.9708, 122.2375)
  line L4573 (121.9708, 103.1875) -> (127.4701, 112.7125)
  line L4574 (141.2182, 133.35) -> (130.2197, 133.35)
  line L4575 (130.2197, 133.35) -> (124.7205, 123.825)
  line L4576 (124.7205, 123.825) -> (130.2197, 114.3)
  line L4577 (130.2197, 114.3) -> (141.2182, 114.3)
  line L4578 (146.7175, 123.825) -> (141.2182, 133.35)
  line L4579 (141.2182, 114.3) -> (146.7175, 123.825)
  line L4580 (160.4657, 144.4625) -> (149.4671, 144.4625)
  line L4581 (149.4671, 144.4625) -> (143.9679, 134.9375)
  line L4582 (143.9679, 134.9375) -> (149.4671, 125.4125)
  line L4583 (149.4671, 125.4125) -> (160.4657, 125.4125)
  line L4584 (165.9649, 134.9375) -> (160.4657, 144.4625)
  line L4585 (160.4657, 125.4125) -> (165.9649, 134.9375)
  line L4586 (179.7131, 155.575) -> (168.7145, 155.575)
  line L4587 (168.7145, 155.575) -> (163.2153, 146.05)
  line L4588 (163.2153, 146.05) -> (168.7145, 136.525)
  line L4589 (168.7145, 136.525) -> (179.7131, 136.525)
  line L4590 (185.2123, 146.05) -> (179.7131, 155.575)
  line L4591 (179.7131, 136.525) -> (185.2123, 146.05)
  line L4592 (198.9605, 166.6875) -> (187.962, 166.6875)
  line L4593 (187.962, 166.6875) -> (182.4627, 157.1625)
  line L4594 (182.4627, 157.1625) -> (187.962, 147.6375)
  line L4595 (187.962, 147.6375) -> (198.9605, 147.6375)
  line L4596 (204.4597, 157.1625) -> (198.9605, 166.6875)
  line L4597 (198.9605, 147.6375) -> (204.4597, 157.1625)
  line L4598 (218.2079, 177.8) -> (207.2094, 177.8)
  line L4599 (207.2094, 177.8) -> (201.7101, 168.275)
  line L4600 (201.7101, 168.275) -> (207.2094, 158.75)
  line L4601 (207.2094, 158.75) -> (218.2079, 158.75)
  line L4602 (223.7072, 168.275) -> (218.2079, 177.8)
  line L4603 (218.2079, 158.75) -> (223.7072, 168.275)
  line L4604 (237.4553, 188.9125) -> (226.4568, 188.9125)
  line L4605 (226.4568, 188.9125) -> (220.9575, 179.3875)
  line L4606 (220.9575, 179.3875) -> (226.4568, 169.8625)
  line L4607 (226.4568, 169.8625) -> (237.4553, 169.8625)
  line L4608 (242.9546, 179.3875) -> (237.4553, 188.9125)
  line L4609 (237.4553, 169.8625) -> (242.9546, 179.3875)
  line L4610 (256.7027, 200.025) -> (245.7042, 200.025)
  line L4611 (245.7042, 200.025) -> (240.2049, 190.5)
  line L4612 (240.2049, 190.5) -> (245.7042, 180.975)
  line L4613 (245.7042, 180.975) -> (256.7027, 180.975)
  line L4614 (262.202, 190.5) -> (256.7027, 200.025)
  line L4615 (256.7027, 180.975) -> (262.202, 190.5)
  line L4616 (275.9501, 211.1375) -> (264.9516, 211.1375)
  line L4617 (264.9516, 211.1375) -> (259.4524, 201.6125)
  line L4618 (259.4524, 201.6125) -> (264.9516, 192.0875)
  line L4619 (264.9516, 192.0875) -> (275.9501, 192.0875)
  line L4620 (281.4494, 201.6125) -> (275.9501, 211.1375)
  line L4621 (275.9501, 192.0875) -> (281.4494, 201.6125)
  line L4622 (295.1976, 222.25) -> (284.199, 222.25)
  line L4623 (284.199, 222.25) -> (278.6998, 212.725)
  line L4624 (278.6998, 212.725) -> (284.199, 203.2)
  line L4625 (284.199, 203.2) -> (295.1976, 203.2)
  line L4626 (300.6968, 212.725) -> (295.1976, 222.25)
  line L4627 (295.1976, 203.2) -> (300.6968, 212.725)
  line L4628 (314.445, 233.3625) -> (303.4464, 233.3625)
  line L4629 (303.4464, 233.3625) -> (297.9472, 223.8375)
  line L4630 (297.9472, 223.8375) -> (303.4464, 214.3125)
  line L4631 (303.4464, 214.3125) -> (314.445, 214.3125)
  line L4632 (319.9442, 223.8375) -> (314.445, 233.3625)
  line L4633 (314.445, 214.3125) -> (319.9442, 223.8375)
  line L4634 (333.6924, 244.475) -> (322.6939, 244.475)
  line L4635 (322.6939, 244.475) -> (317.1946, 234.95)
  line L4636 (317.1946, 234.95) -> (322.6939, 225.425)
  line L4637 (322.6939, 225.425) -> (333.6924, 225.425)
  line L4638 (339.1916, 234.95) -> (333.6924, 244.475)
  line L4639 (333.6924, 225.425) -> (339.1916, 234.95)
  line L4640 (352.9398, 255.5875) -> (341.9413, 255.5875)
  line L4641 (341.9413, 255.5875) -> (336.442, 246.0625)
  line L4642 (336.442, 246.0625) -> (341.9413, 236.5375)
  line L4643 (341.9413, 236.5375) -> (352.9398, 236.5375)
  line L4644 (358.4391, 246.0625) -> (352.9398, 255.5875)
  line L4645 (352.9398, 236.5375) -> (358.4391, 246.0625)
  line L4646 (372.1872, 266.7) -> (361.1887, 266.7)
  line L4647 (361.1887, 266.7) -> (355.6894, 257.175)
  line L4648 (355.6894, 257.175) -> (361.1887, 247.65)
  line L4649 (361.1887, 247.65) -> (372.1872, 247.65)
  line L4650 (377.6865, 257.175) -> (372.1872, 266.7)
  line L4651 (372.1872, 247.65) -> (377.6865, 257.175)
  line L4652 (391.4346, 277.8125) -> (380.4361, 277.8125)
  line L4653 (380.4361, 277.8125) -> (374.9368, 268.2875)
  line L4654 (374.9368, 268.2875) -> (380.4361, 258.7625)
  line L4655 (380.4361, 258.7625) -> (391.4346, 258.7625)
  line L4656 (396.9339, 268.2875) -> (391.4346, 277.8125)
  line L4657 (391.4346, 258.7625) -> (396.9339, 268.2875)
  line L4658 (410.682, 288.925) -> (399.6835, 288.925)
  line L4659 (399.6835, 288.925) -> (394.1843, 279.4)
  line L4660 (394.1843, 279.4) -> (399.6835, 269.875)
  line L4661 (399.6835, 269.875) -> (410.682, 269.875)
  line L4662 (416.1813, 279.4) -> (410.682, 288.925)
  line L4663 (410.682, 269.875) -> (416.1813, 279.4)
  line L4664 (429.9295, 300.0375) -> (418.9309, 300.0375)
  line L4665 (418.9309, 300.0375) -> (413.4317, 290.5125)
  line L4666 (413.4317, 290.5125) -> (418.9309, 280.9875)
  line L4667 (418.9309, 280.9875) -> (429.9295, 280.9875)
  line L4668 (435.4287, 290.5125) -> (429.9295, 300.0375)
  line L4669 (429.9295, 280.9875) -> (435.4287, 290.5125)
  line L4670 (449.1769, 311.15) -> (438.1783, 311.15)
  line L4671 (438.1783, 311.15) -> (432.6791, 301.625)
  line L4672 (432.6791, 301.625) -> (438.1783, 292.1)
  line L4673 (438.1783, 292.1) -> (449.1769, 292.1)
  line L4674 (454.6761, 301.625) -> (449.1769, 311.15)
  line L4675 (449.1769, 292.1) -> (454.6761, 301.625)
  line L4676 (468.4243, 322.2625) -> (457.4258, 322.2625)
  line L4677 (457.4258, 322.2625) -> (451.9265, 312.7375)
  line L4678 (451.9265, 312.7375) -> (457.4258, 303.2125)
  line L4679 (457.4258, 303.2125) -> (468.4243, 303.2125)
  line L4680 (473.9235, 312.7375) -> (468.4243, 322.2625)
  line L4681 (468.4243, 303.2125) -> (473.9235, 312.7375)
  line L4682 (487.6717, 333.375) -> (476.6732, 333.375)
  line L4683 (476.6732, 333.375) -> (471.1739, 323.85)
  line L4684 (471.1739, 323.85) -> (476.6732, 314.325)
  line L4685 (476.6732, 314.325) -> (487.6717, 314.325)
  line L4686 (493.171, 323.85) -> (487.6717, 333.375)
  line L4687 (487.6717, 314.325) -> (493.171, 323.85)
  line L4688 (506.9191, 344.4875) -> (495.9206, 344.4875)
  line L4689 (495.9206, 344.4875) -> (490.4213, 334.9625)
  line L4690 (490.4213, 334.9625) -> (495.9206, 325.4375)
  line L4691 (495.9206, 325.4375) -> (506.9191, 325.4375)
  line L4692 (512.4184, 334.9625) -> (506.9191, 344.4875)
  line L4693 (506.9191, 325.4375) -> (512.4184, 334.9625)
  line L4694 (526.1665, 355.6) -> (515.168, 355.6)
  line L4695 (515.168, 355.6) -> (509.6687, 346.075)
  line L4696 (509.6687, 346.075) -> (515.168, 336.55)
  line L4697 (515.168, 336.55) -> (526.1665, 336.55)
  line L4698 (531.6658, 346.075) -> (526.1665, 355.6)
  line L4699 (526.1665, 336.55) -> (531.6658, 346.075)
  line L4700 (-628.6783, -288.925) -> (-639.6769, -288.925)
  line L4701 (-639.6769, -288.925) -> (-645.1761, -298.45)
  line L4702 (-645.1761, -298.45) -> (-639.6769, -307.975)
  line L4703 (-639.6769, -307.975) -> (-628.6783, -307.975)
  line L4704 (-623.1791, -298.45) -> (-628.6783, -288.925)
  line L4705 (-628.6783, -307.975) -> (-623.1791, -298.45)
  line L4706 (-609.4309, -277.8125) -> (-620.4295, -277.8125)
  line L4707 (-620.4295, -277.8125) -> (-625.9287, -287.3375)
  line L4708 (-625.9287, -287.3375) -> (-620.4295, -296.8625)
  line L4709 (-620.4295, -296.8625) -> (-609.4309, -296.8625)
  line L4710 (-603.9317, -287.3375) -> (-609.4309, -277.8125)
  line L4711 (-609.4309, -296.8625) -> (-603.9317, -287.3375)
  line L4712 (-590.1835, -266.7) -> (-601.182, -266.7)
  line L4713 (-601.182, -266.7) -> (-606.6813, -276.225)
  line L4714 (-606.6813, -276.225) -> (-601.182, -285.75)
  line L4715 (-601.182, -285.75) -> (-590.1835, -285.75)
  line L4716 (-584.6843, -276.225) -> (-590.1835, -266.7)
  line L4717 (-590.1835, -285.75) -> (-584.6843, -276.225)
  line L4718 (-570.9361, -255.5875) -> (-581.9346, -255.5875)
  line L4719 (-581.9346, -255.5875) -> (-587.4339, -265.1125)
  line L4720 (-587.4339, -265.1125) -> (-581.9346, -274.6375)
  line L4721 (-581.9346, -274.6375) -> (-570.9361, -274.6375)
  line L4722 (-565.4368, -265.1125) -> (-570.9361, -255.5875)
  line L4723 (-570.9361, -274.6375) -> (-565.4368, -265.1125)
  line L4724 (-551.6887, -244.475) -> (-562.6872, -244.475)
  line L4725 (-562.6872, -244.475) -> (-568.1865, -254)
  line L4726 (-568.1865, -254) -> (-562.6872, -263.525)
  line L4727 (-562.6872, -263.525) -> (-551.6887, -263.525)
  line L4728 (-546.1894, -254) -> (-551.6887, -244.475)
  line L4729 (-551.6887, -263.525) -> (-546.1894, -254)
  line L4730 (-532.4413, -233.3625) -> (-543.4398, -233.3625)
  line L4731 (-543.4398, -233.3625) -> (-548.9391, -242.8875)
  line L4732 (-548.9391, -242.8875) -> (-543.4398, -252.4125)
  line L4733 (-543.4398, -252.4125) -> (-532.4413, -252.4125)
  line L4734 (-526.942, -242.8875) -> (-532.4413, -233.3625)
  line L4735 (-532.4413, -252.4125) -> (-526.942, -242.8875)
  line L4736 (-513.1939, -222.25) -> (-524.1924, -222.25)
  line L4737 (-524.1924, -222.25) -> (-529.6916, -231.775)
  line L4738 (-529.6916, -231.775) -> (-524.1924, -241.3)
  line L4739 (-524.1924, -241.3) -> (-513.1939, -241.3)
  line L4740 (-507.6946, -231.775) -> (-513.1939, -222.25)
  line L4741 (-513.1939, -241.3) -> (-507.6946, -231.775)
  line L4742 (-493.9464, -211.1375) -> (-504.945, -211.1375)
  line L4743 (-504.945, -211.1375) -> (-510.4442, -220.6625)
  line L4744 (-510.4442, -220.6625) -> (-504.945, -230.1875)
  line L4745 (-504.945, -230.1875) -> (-493.9464, -230.1875)